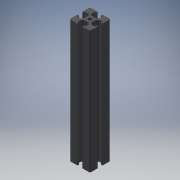
# Autodesk Inventor part: HFS3-1515-90
Saved by Autodesk Inventor 2016 (Build 200138000, 138)
## iProperties
Category: PARTsolutions
Company: MISUMI
Created: 2016-11-23
Part Number: HFS3-1515-90
Catalog Web Link: www.cadenas.de
Description: HFS3, KHFS3-Aluminum Frames 15mm Square
Vendor: MISUMI
Document SubType Name: Modeling
Designer: psAdmin
Manufacturer: MISUMI
Mass: 11.2873 g
Surface Area: 107.866 cm^2
Volume: 11.2873 cm^3
Density: 1 g/cm^3
Material: 一般
Appearance: PSOLRGB-175-175-175
PSOL_IDENT_0: {$CADENAS_DATA\23d-libs\misumi\metric\38_al_extrusions_blackets\hfs3_1515.prj},172 {VTYP=3D},{NB=HFS
PSOL_IDENT_1: 3-1515-90},{LINA=HFS3-1515-90},{NN=HFS3, KHFS3},{DATE=17.06.2016 05:53:31},{GEOMDATE=07.03.2008 00:0
PSOL_IDENT_2: 0:00},{VERSION=},{LINEID=10},{LINESUBID=-1},{WBVAR=L}  {NB=HFS3-1515-90},{LINA=HFS3-1515-90},{KT=LIN
PSOL_IDENT_3: A},{PN=HFS3-1515-90},{MAT=A6N01SS-T5(Aluminum)(EN AC-51400_AlMgSiO,7-T5)},{ST=Alumite},{LT=Specified
PSOL_IDENT_4: Length},{L=90.0},{FEAT=4 Slots},{LALG=[50-2000/0.5]},{LTOL=+/- 0.5},{MASS=0.34},{SA=126},{SMILX=0.2
PSOL_IDENT_5: 80x10^4},{SMILY=0.280x10^4},{TYPE=HFS3-1515}
NN: HFS3, KHFS3
NT: Aluminum Frames 15mm Square
NB: HFS3-1515-90
NBSYN: $PN.
LINA: HFS3-1515-90
PN: HFS3-1515-90
MAT: A6N01SS-T5
ST: Clear Anodizing
LT: Specified Length
L: 90.0
LTOL: +/- 0.5
MASS: 0.34
SA: 126
SMILX: 0.280x10^4
SMILY: 0.280x10^4
SUPPLIER: MISUMI
ARTICLENO: HFS3-1515-90
BOMINFO: HFS3-1515-90
CREATOR: CADENAS GmbH
Title: HFS3-1515-90
Author: Cadenas PARTsolutions
Comments: Aluminum Frames 15mm Square
Autodesk Inventor part; units mm, degrees
ref_plane "YZ Plane" through (0, 0, 0) normal (1, 0, 0) x (0, 1, 0)
ref_plane "XZ Plane" through (0, 0, 0) normal (0, 1, 0) x (-1, 0, 0)
ref_plane "XY Plane" through (0, 0, 0) normal (0, 0, 1) x (1, 0, 0)
sketch "Sketch_1" plane through (0, 0, 0) normal (0, 0, 1) x (1, 0, 0)
  line L0 (-7.5, 6.5) -> (-7.5, 2)
  arc A0 (-7.5, 2) -> (-7.2, 1.7) centre (-7.2, 2) ccw
  line L1 (-7.2, 1.7) -> (-6.4, 1.7)
  line L2 (-6.4, 1.7) -> (-6.4, 2.85)
  line L3 (-6.4, 2.85) -> (-3.8, 2.85)
  line L4 (-3.8, 2.85) -> (-2.8, 1.85)
  line L5 (-2.8, 1.85) -> (-2.8, 0.5196)
  line L6 (-2.8, 0.5196) -> (-2.5, 0)
  line L7 (-2.5, 0) -> (-2.8, -0.5196)
  line L8 (-2.8, -0.5196) -> (-2.8, -1.85)
  line L9 (-2.8, -1.85) -> (-3.8, -2.85)
  line L10 (-3.8, -2.85) -> (-6.4, -2.85)
  line L11 (-6.4, -2.85) -> (-6.4, -1.7)
  line L12 (-6.4, -1.7) -> (-7.2, -1.7)
  arc A1 (-7.2, -1.7) -> (-7.5, -2) centre (-7.2, -2) ccw
  line L13 (-7.5, -2) -> (-7.5, -6.5)
  arc A2 (-7.5, -6.5) -> (-6.5, -7.5) centre (-6.5, -6.5) ccw
  line L14 (-6.5, -7.5) -> (-2, -7.5)
  arc A3 (-2, -7.5) -> (-1.7, -7.2) centre (-2, -7.2) ccw
  line L15 (-1.7, -7.2) -> (-1.7, -6.4)
  line L16 (-1.7, -6.4) -> (-2.85, -6.4)
  line L17 (-2.85, -6.4) -> (-2.85, -3.8)
  line L18 (-2.85, -3.8) -> (-1.85, -2.8)
  line L19 (-1.85, -2.8) -> (-0.5196, -2.8)
  line L20 (-0.5196, -2.8) -> (0, -2.5)
  line L21 (0, -2.5) -> (0.5196, -2.8)
  line L22 (0.5196, -2.8) -> (1.85, -2.8)
  line L23 (1.85, -2.8) -> (2.85, -3.8)
  line L24 (2.85, -3.8) -> (2.85, -6.4)
  line L25 (2.85, -6.4) -> (1.7, -6.4)
  line L26 (1.7, -6.4) -> (1.7, -7.2)
  arc A4 (1.7, -7.2) -> (2, -7.5) centre (2, -7.2) ccw
  line L27 (2, -7.5) -> (6.5, -7.5)
  arc A5 (6.5, -7.5) -> (7.5, -6.5) centre (6.5, -6.5) ccw
  line L28 (7.5, -6.5) -> (7.5, -2)
  arc A6 (7.5, -2) -> (7.2, -1.7) centre (7.2, -2) ccw
  line L29 (7.2, -1.7) -> (6.4, -1.7)
  line L30 (6.4, -1.7) -> (6.4, -2.85)
  line L31 (6.4, -2.85) -> (3.8, -2.85)
  line L32 (3.8, -2.85) -> (2.8, -1.85)
  line L33 (2.8, -1.85) -> (2.8, -0.5196)
  line L34 (2.8, -0.5196) -> (2.5, 0)
  line L35 (2.5, 0) -> (2.8, 0.5196)
  line L36 (2.8, 0.5196) -> (2.8, 1.85)
  line L37 (2.8, 1.85) -> (3.8, 2.85)
  line L38 (3.8, 2.85) -> (6.4, 2.85)
  line L39 (6.4, 2.85) -> (6.4, 1.7)
  line L40 (6.4, 1.7) -> (7.2, 1.7)
  arc A7 (7.2, 1.7) -> (7.5, 2) centre (7.2, 2) ccw
  line L41 (7.5, 2) -> (7.5, 6.5)
  arc A8 (7.5, 6.5) -> (6.5, 7.5) centre (6.5, 6.5) ccw
  line L42 (6.5, 7.5) -> (2, 7.5)
  arc A9 (2, 7.5) -> (1.7, 7.2) centre (2, 7.2) ccw
  line L43 (1.7, 7.2) -> (1.7, 6.4)
  line L44 (1.7, 6.4) -> (2.85, 6.4)
  line L45 (2.85, 6.4) -> (2.85, 3.8)
  line L46 (2.85, 3.8) -> (1.85, 2.8)
  line L47 (1.85, 2.8) -> (0.5196, 2.8)
  line L48 (0.5196, 2.8) -> (0, 2.5)
  line L49 (0, 2.5) -> (-0.5196, 2.8)
  line L50 (-0.5196, 2.8) -> (-1.85, 2.8)
  line L51 (-1.85, 2.8) -> (-2.85, 3.8)
  line L52 (-2.85, 3.8) -> (-2.85, 6.4)
  line L53 (-2.85, 6.4) -> (-1.7, 6.4)
  line L54 (-1.7, 6.4) -> (-1.7, 7.2)
  arc A10 (-1.7, 7.2) -> (-2, 7.5) centre (-2, 7.2) ccw
  line L55 (-2, 7.5) -> (-6.5, 7.5)
  arc A11 (-6.5, 7.5) -> (-7.5, 6.5) centre (-6.5, 6.5) ccw
  circle A12 centre (0, 0) radius 1.25
  constraints: 112 end point, 24 point on circle, 13 centre point
extrude "Extrusion1" add sketch "Sketch_1" along normal blind 90
body "Solid1"
